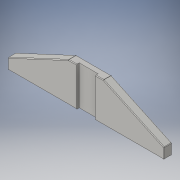
# Autodesk Inventor part: Foot
Saved by Autodesk Inventor 2016 (Build 200138000, 138)
## iProperties
Created: 2016-07-05
Part Number: Foot
Material: Generic
Document SubType Name: Modeling
Designer: kurti
Density: 1 g/cm^3
Appearance: Default
Author: kurti
Autodesk Inventor part; units mm, degrees
ref_plane "YZ Plane" through (0, 0, 0) normal (1, 0, 0) x (0, 1, 0)
ref_plane "XZ Plane" through (0, 0, 0) normal (0, 1, 0) x (-1, 0, 0)
ref_plane "XY Plane" through (0, 0, 0) normal (0, 0, 1) x (1, 0, 0)
sketch "Sketch1" plane through (0, 0, 0) normal (0, 0, 1) x (1, 0, 0)
  line L0 (0, 0) -> (736.6, 0)
  line L1 (368.3, 0) -> (368.3, 184.15) construction
  line L2 (368.3, 184.15) -> (450.85, 184.15)
  line L3 (368.3, 184.15) -> (285.75, 184.15)
  line L4 (0, 0) -> (0, 50.8)
  line L5 (736.6, 0) -> (736.6, 50.8)
  line L6 (736.6, 50.8) -> (450.85, 184.15)
  line L7 (0, 50.8) -> (285.75, 184.15)
  dimension "d0" = 736.6
  dimension "d1" = 184.15
  dimension "d2" = 82.55
  dimension "d3" = 82.55
  dimension "d4" = 50.8
  dimension "d5" = 50.8
  constraints: 16 end point, 3 vertical, 2 horizontal, 1 midpoint, 1 perpendicular
  measures "d0" distance of L0.start L0.end
  measures "d1" distance of L1.start L1.end
  measures "d2" distance of L1.end L2.end
  measures "d3" distance of L1.end L3.end
  measures "d4" distance of L0.start L4.end
  measures "d5" distance of L0.end L5.end
extrude "Extrusion1" add sketch "Sketch1" along normal blind 38.1
sketch "Sketch2" plane through (285.75, 184.15, 0) normal (0, 1, 0) x (1, 0, 0)
  line L0 (38.1, -50.8) -> (127, -50.8)
  line L1 (127, -50.8) -> (127, -25.4)
  line L2 (127, -25.4) -> (38.1, -25.4)
  line L3 (38.1, -25.4) -> (38.1, -50.8)
  line L4 (-285.75, -38.1) -> (450.85, -38.1) projected
  line L5 (38.1, -50.8) -> (127, -25.4) construction
  line L6 (127, -50.8) -> (38.1, -25.4) construction
  point P0 (-285.75, 0)
  point P1 (82.55, -38.1)
  dimension "d8" = 88.9
  dimension "d9" = 25.4
  constraints: 12 end point, 3 midpoint, 2 parallel, 1 horizontal, 1 perpendicular
  measures "d8" distance of L2.end L1.end
  measures "d9" distance of L1.end L0.end
extrude "Extrusion2" cut sketch "Sketch2" against normal blind 184.15
fillet "Fillet1" radius 3.175 20 edges at (142.875, 117.475, 38.1) (142.875, 117.475, 0) (368.3, 184.15, 0) (593.725, 117.475, 0) (593.725, 117.475, 38.1) (0, 50.8, 19.05) (285.75, 184.15, 19.05) (450.85, 184.15, 19.05) (736.6, 50.8, 19.05) (736.6, 25.4, 0) (736.6, 0, 19.05) (736.6, 25.4, 38.1) (368.3, 0, 0) (574.675, 0, 38.1) (0, 0, 19.05) (0, 25.4, 0) (0, 25.4, 38.1) (161.925, 0, 38.1) (431.8, 184.15, 38.1) (304.8, 184.15, 38.1)
body "Solid1"
